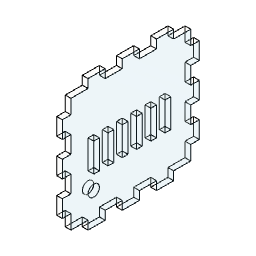
case_3_3mm (Autodesk Fusion 360 design; units mm, degrees)
Autodesk Fusion 360 part; units mm, degrees
sketch "スケッチ1" plane through (0, 0, 0) normal (1, 0, 0) x (0, 1, 0)
  line L0 (0, 0) -> (46, 0)
  line L1 (46, 0) -> (46, 44)
  line L2 (46, 44) -> (0, 44)
  line L3 (0, 44) -> (0, 0)
  dimension "d1" = 46
  dimension "d2" = 44
  constraint horizontal L0
  constraint vertical L1
  constraint horizontal L2
  constraint vertical L3
  constraint coincident L0.start L3.end
  measures "d1" distance of L0.start L0.end
  measures "d2" distance of L0.end L1.end
extrude "押し出し1" add sketch "スケッチ1" along normal blind 2
sketch "スケッチ2" plane through (2, 0, 0) normal (1, 0, 0) x (0, 1, 0)
  line L0 (0, 44) -> (0, 0)
  line L1 (0, 0) -> (46, 0)
  line L2 (46, 0) -> (46, 44)
  line L3 (46, 44) -> (0, 44)
  line L4 (0, 0) -> (8, 0)
  line L5 (8, 0) -> (8, 2)
  line L6 (8, 2) -> (0, 2)
  line L7 (0, 2) -> (0, 0)
  line L8 (14, 0) -> (20, 0)
  line L9 (20, 0) -> (20, 2)
  line L10 (20, 2) -> (14, 2)
  line L11 (14, 2) -> (14, 0)
  line L12 (26, 0) -> (32, 0)
  line L13 (32, 0) -> (32, 2)
  line L14 (32, 2) -> (26, 2)
  line L15 (26, 2) -> (26, 0)
  line L16 (46, 0) -> (38, 0)
  line L17 (38, 0) -> (38, 2)
  line L18 (38, 2) -> (46, 2)
  line L19 (46, 2) -> (46, 0)
  line L20 (32, 42) -> (32, 44)
  line L21 (32, 44) -> (26, 44)
  line L22 (20, 42) -> (20, 44)
  line L23 (38, 42) -> (38, 44)
  line L24 (38, 44) -> (46, 44)
  line L25 (46, 44) -> (46, 42)
  line L26 (0, 42) -> (8, 42)
  line L27 (26, 44) -> (26, 42)
  line L28 (8, 42) -> (8, 44)
  line L29 (8, 44) -> (0, 44)
  line L30 (0, 44) -> (0, 42)
  line L31 (20, 44) -> (14, 44)
  line L32 (26, 42) -> (32, 42)
  line L33 (46, 42) -> (38, 42)
  line L34 (14, 42) -> (20, 42)
  line L35 (14, 44) -> (14, 42)
  point P0 (0, 42)
  dimension "d5" = 8
  dimension "d6" = 2
  dimension "d7" = 6
  dimension "d8" = 2
  dimension "d9" = 6
  dimension "d10" = 6
  dimension "d11" = 2
  dimension "d12" = 6
  dimension "d13" = 6
  dimension "d14" = 2
  constraint horizontal L4
  constraint vertical L5
  constraint horizontal L6
  constraint vertical L7
  constraint coincident L0.end L1.start
  constraint horizontal L8
  constraint vertical L9
  constraint horizontal L10
  constraint vertical L11
  constraint coincident L1 L8.start
  constraint horizontal L12
  constraint vertical L13
  constraint horizontal L14
  constraint vertical L15
  constraint coincident L1 L12.start
  constraint horizontal L16
  constraint vertical L17
  constraint horizontal L18
  constraint vertical L19
  constraint coincident L1.end L2.start
  measures "d5" distance of L5.end L6.end
  measures "d6" distance of L0.end L6.end
  measures "d7" distance of L9.end L10.end
  measures "d8" distance of L8.start L10.end
  measures "d9" distance of L5 L11
  measures "d10" distance of L13.end L14.end
  measures "d11" distance of L12.start L14.end
  measures "d12" distance of L9 L15
  measures "d13" distance of L13 L17
  measures "d14" distance of L1.end L18.end
extrude "押し出し2" cut sketch "スケッチ2" against normal blind 2 contours L0 L3 L26 L28 L29 L30 | L0 L1 L4 L5 L6 L7 | L3 L22 L31 L34 L35 | L3 L20 L21 L27 L32 | L1 L8 L9 L10 L11 | L2 L3 L23 L24 L25 L33 | L1 L12 L13 L14 L15 | L1 L2 L16 L17 L18 L19
sketch "スケッチ3" plane through (2, 0, 0) normal (1, 0, 0) x (0, 1, 0)
  line L0 (8, 2) -> (8, 0)
  line L1 (8, 0) -> (14, 0)
  line L2 (14, 0) -> (14, 2)
  line L3 (14, 2) -> (20, 2)
  line L4 (20, 2) -> (20, 0)
  line L5 (20, 0) -> (26, 0)
  line L6 (26, 0) -> (26, 2)
  line L7 (26, 2) -> (32, 2)
  line L8 (32, 2) -> (32, 0)
  line L9 (32, 0) -> (38, 0)
  line L10 (38, 0) -> (38, 2)
  line L11 (38, 2) -> (46, 2)
  line L12 (46, 2) -> (46, 42)
  line L13 (46, 42) -> (38, 42)
  line L14 (38, 42) -> (38, 44)
  line L15 (38, 44) -> (32, 44)
  line L16 (32, 44) -> (32, 42)
  line L17 (32, 42) -> (26, 42)
  line L18 (26, 42) -> (26, 44)
  line L19 (26, 44) -> (20, 44)
  line L20 (20, 44) -> (20, 42)
  line L21 (20, 42) -> (14, 42)
  line L22 (14, 42) -> (14, 44)
  line L23 (14, 44) -> (8, 44)
  line L24 (8, 44) -> (8, 42)
  line L25 (8, 42) -> (0, 42)
  line L26 (0, 42) -> (0, 2)
  line L27 (0, 2) -> (8, 2)
  line L28 (0, 44) -> (2, 44)
  line L29 (2, 44) -> (2, 37)
  line L30 (2, 37) -> (0, 37)
  line L31 (0, 37) -> (0, 44)
  line L32 (2, 31) -> (0, 31)
  line L33 (0, 31) -> (0, 25)
  line L34 (0, 25) -> (2, 25)
  line L35 (2, 25) -> (2, 31)
  line L36 (2, 19) -> (0, 19)
  line L37 (0, 19) -> (0, 13)
  line L38 (0, 13) -> (2, 13)
  line L39 (2, 13) -> (2, 19)
  line L40 (2, 7) -> (0, 7)
  line L41 (0, 7) -> (0, 0)
  line L42 (0, 0) -> (2, 0)
  line L43 (2, 0) -> (2, 7)
  line L44 (46, 31) -> (44, 31)
  line L45 (46, 13) -> (46, 19)
  line L46 (44, 44) -> (46, 44)
  line L47 (44, 0) -> (46, 0)
  line L48 (44, 7) -> (44, 0)
  line L49 (44, 25) -> (46, 25)
  line L50 (46, 37) -> (44, 37)
  line L51 (44, 37) -> (44, 44)
  line L52 (44, 13) -> (46, 13)
  line L53 (44, 31) -> (44, 25)
  line L54 (46, 19) -> (44, 19)
  line L55 (44, 19) -> (44, 13)
  line L56 (46, 25) -> (46, 31)
  line L57 (46, 7) -> (44, 7)
  line L58 (46, 0) -> (46, 7)
  line L59 (46, 44) -> (46, 37)
  point P0 (44, 0)
  dimension "d21" = 2
  dimension "d22" = 7
  dimension "d23" = 2
  dimension "d24" = 6
  dimension "d25" = 6
  dimension "d26" = 6
  dimension "d27" = 6
  dimension "d28" = 2
  dimension "d29" = 6
  dimension "d30" = 7
  dimension "d31" = 2
  constraint horizontal L28
  constraint vertical L29
  constraint horizontal L30
  constraint vertical L31
  constraint horizontal L32
  constraint vertical L33
  constraint horizontal L34
  constraint vertical L35
  constraint coincident L26 L33.end
  constraint horizontal L36
  constraint vertical L37
  constraint horizontal L38
  constraint vertical L39
  constraint coincident L26 L37.end
  constraint horizontal L40
  constraint vertical L41
  constraint horizontal L42
  constraint vertical L43
  constraint coincident L41.end L42.start
  measures "d21" distance of L28.start L28.end
  measures "d22" distance of L28.start L30.end
  measures "d23" distance of L32.start L32.end
  measures "d24" distance of L32.end L33.end
  measures "d25" distance of L30 L32
  measures "d26" distance of L34 L36
  measures "d27" distance of L36.end L37.end
  measures "d28" distance of L36.start L36.end
  measures "d29" distance of L38 L40
  measures "d30" distance of L40.end L41.end
  measures "d31" distance of L40.start L40.end
extrude "押し出し3" cut sketch "スケッチ3" against normal blind 2 contours L27 L41 L42 L43 | L26 L27 L40 L41 L43 | L26 L36 L37 L38 L39 | L26 L32 L33 L34 L35 | L25 L26 L29 L30 L31 | L25 L28 L29 L31 | L11 L12 L48 L57 L58 | L11 L47 L48 L58 | L12 L45 L52 L54 L55 | L12 L44 L49 L53 L56 | L12 L13 L50 L51 L59 | L13 L46 L51 L59
sketch "スケッチ4" plane through (2, 0, 0) normal (1, 0, 0) x (0, 1, 0)
  line L0 (44, 19) -> (46, 19)
  line L1 (46, 19) -> (46, 25)
  line L2 (46, 25) -> (44, 25)
  line L3 (44, 25) -> (44, 31)
  line L4 (44, 31) -> (46, 31)
  line L5 (46, 31) -> (46, 37)
  line L6 (46, 37) -> (44, 37)
  line L7 (44, 37) -> (44, 42)
  line L8 (44, 42) -> (38, 42)
  line L9 (38, 42) -> (38, 44)
  line L10 (38, 44) -> (32, 44)
  line L11 (32, 44) -> (32, 42)
  line L12 (32, 42) -> (26, 42)
  line L13 (26, 42) -> (26, 44)
  line L14 (26, 44) -> (20, 44)
  line L15 (20, 44) -> (20, 42)
  line L16 (20, 42) -> (14, 42)
  line L17 (14, 42) -> (14, 44)
  line L18 (14, 44) -> (8, 44)
  line L19 (8, 44) -> (8, 42)
  line L20 (8, 42) -> (2, 42)
  line L21 (2, 42) -> (2, 37)
  line L22 (2, 37) -> (0, 37)
  line L23 (0, 37) -> (0, 31)
  line L24 (0, 31) -> (2, 31)
  line L25 (2, 31) -> (2, 25)
  line L26 (2, 25) -> (0, 25)
  line L27 (0, 25) -> (0, 19)
  line L28 (0, 19) -> (2, 19)
  line L29 (2, 19) -> (2, 13)
  line L30 (2, 13) -> (0, 13)
  line L31 (0, 13) -> (0, 7)
  line L32 (0, 7) -> (2, 7)
  line L33 (2, 7) -> (2, 2)
  line L34 (2, 2) -> (8, 2)
  line L35 (8, 2) -> (8, 0)
  line L36 (8, 0) -> (14, 0)
  line L37 (14, 0) -> (14, 2)
  line L38 (14, 2) -> (20, 2)
  line L39 (20, 2) -> (20, 0)
  line L40 (20, 0) -> (26, 0)
  line L41 (26, 0) -> (26, 2)
  line L42 (26, 2) -> (32, 2)
  line L43 (32, 2) -> (32, 0)
  line L44 (32, 0) -> (38, 0)
  line L45 (38, 0) -> (38, 2)
  line L46 (38, 2) -> (44, 2)
  line L47 (44, 2) -> (44, 7)
  line L48 (44, 7) -> (46, 7)
  line L49 (46, 7) -> (46, 13)
  line L50 (46, 13) -> (44, 13)
  line L51 (44, 13) -> (44, 19)
  line L52 (10, 15) -> (12, 15)
  line L53 (12, 15) -> (12, 25)
  line L54 (12, 25) -> (10, 25)
  line L55 (10, 25) -> (10, 15)
  line L56 (15, 15) -> (17, 15)
  line L57 (17, 15) -> (17, 25)
  line L58 (17, 25) -> (15, 25)
  line L59 (15, 25) -> (15, 15)
  line L60 (20, 15) -> (22, 15)
  line L61 (22, 15) -> (22, 25)
  line L62 (22, 25) -> (20, 25)
  line L63 (20, 25) -> (20, 15)
  line L64 (25, 15) -> (27, 15)
  line L65 (27, 15) -> (27, 25)
  line L66 (27, 25) -> (25, 25)
  line L67 (25, 25) -> (25, 15)
  line L68 (30, 15) -> (32, 15)
  line L69 (32, 15) -> (32, 25)
  line L70 (32, 25) -> (30, 25)
  line L71 (30, 25) -> (30, 15)
  line L72 (35, 15) -> (37, 15)
  line L73 (37, 15) -> (37, 25)
  line L74 (37, 25) -> (35, 25)
  line L75 (35, 25) -> (35, 15)
  constraint horizontal L52
  constraint vertical L53
  constraint horizontal L54
  constraint vertical L55
  constraint horizontal L56
  constraint vertical L57
  constraint horizontal L58
  constraint vertical L59
  constraint horizontal L60
  constraint vertical L61
  constraint horizontal L62
  constraint vertical L63
  constraint horizontal L64
  constraint vertical L65
  constraint horizontal L66
  constraint vertical L67
  constraint horizontal L68
  constraint vertical L69
  constraint horizontal L70
  constraint vertical L71
  constraint horizontal L72
  constraint vertical L73
  constraint horizontal L74
  constraint vertical L75
extrude "押し出し4" cut sketch "スケッチ4" against normal blind 2 contours L52 L53 L54 L55 | L56 L57 L58 L59 | L60 L61 L62 L63 | L64 L65 L66 L67 | L68 L69 L70 L71 | L72 L73 L74 L75
sketch "スケッチ5" plane through (2, 0, 0) normal (1, 0, 0) x (0, 1, 0)
  line L0 (37, 15) -> (35, 15)
  line L1 (35, 15) -> (35, 25)
  line L2 (35, 25) -> (37, 25)
  line L3 (37, 25) -> (37, 15)
  line L4 (32, 15) -> (30, 15)
  line L5 (30, 15) -> (30, 25)
  line L6 (30, 25) -> (32, 25)
  line L7 (32, 25) -> (32, 15)
  line L8 (17, 15) -> (15, 15)
  line L9 (15, 15) -> (15, 25)
  line L10 (15, 25) -> (17, 25)
  line L11 (17, 25) -> (17, 15)
  line L12 (12, 15) -> (10, 15)
  line L13 (10, 15) -> (10, 25)
  line L14 (10, 25) -> (12, 25)
  line L15 (12, 25) -> (12, 15)
  line L16 (22, 15) -> (20, 15)
  line L17 (20, 15) -> (20, 25)
  line L18 (20, 25) -> (22, 25)
  line L19 (22, 25) -> (22, 15)
  line L20 (27, 15) -> (25, 15)
  line L21 (25, 15) -> (25, 25)
  line L22 (25, 25) -> (27, 25)
  line L23 (27, 25) -> (27, 15)
  line L24 (44, 19) -> (46, 19)
  line L25 (46, 19) -> (46, 25)
  line L26 (46, 25) -> (44, 25)
  line L27 (44, 25) -> (44, 31)
  line L28 (44, 31) -> (46, 31)
  line L29 (46, 31) -> (46, 37)
  line L30 (46, 37) -> (44, 37)
  line L31 (44, 37) -> (44, 42)
  line L32 (44, 42) -> (38, 42)
  line L33 (38, 42) -> (38, 44)
  line L34 (38, 44) -> (32, 44)
  line L35 (32, 44) -> (32, 42)
  line L36 (32, 42) -> (26, 42)
  line L37 (26, 42) -> (26, 44)
  line L38 (26, 44) -> (20, 44)
  line L39 (20, 44) -> (20, 42)
  line L40 (20, 42) -> (14, 42)
  line L41 (14, 42) -> (14, 44)
  line L42 (14, 44) -> (8, 44)
  line L43 (8, 44) -> (8, 42)
  line L44 (8, 42) -> (2, 42)
  line L45 (2, 42) -> (2, 37)
  line L46 (2, 37) -> (0, 37)
  line L47 (0, 37) -> (0, 31)
  line L48 (0, 31) -> (2, 31)
  line L49 (2, 31) -> (2, 25)
  line L50 (2, 25) -> (0, 25)
  line L51 (0, 25) -> (0, 19)
  line L52 (0, 19) -> (2, 19)
  line L53 (2, 19) -> (2, 13)
  line L54 (2, 13) -> (0, 13)
  line L55 (0, 13) -> (0, 7)
  line L56 (0, 7) -> (2, 7)
  line L57 (2, 7) -> (2, 2)
  line L58 (2, 2) -> (8, 2)
  line L59 (8, 2) -> (8, 0)
  line L60 (8, 0) -> (14, 0)
  line L61 (14, 0) -> (14, 2)
  line L62 (14, 2) -> (20, 2)
  line L63 (20, 2) -> (20, 0)
  line L64 (20, 0) -> (26, 0)
  line L65 (26, 0) -> (26, 2)
  line L66 (26, 2) -> (32, 2)
  line L67 (32, 2) -> (32, 0)
  line L68 (32, 0) -> (38, 0)
  line L69 (38, 0) -> (38, 2)
  line L70 (38, 2) -> (44, 2)
  line L71 (44, 2) -> (44, 7)
  line L72 (44, 7) -> (46, 7)
  line L73 (46, 7) -> (46, 13)
  line L74 (46, 13) -> (44, 13)
  line L75 (44, 13) -> (44, 19)
  circle A0 centre (10, 10) radius 2
extrude "押し出し5" cut sketch "スケッチ5" against normal blind 2 contours A0
sketch "スケッチ6" plane through (2, 0, 0) normal (1, 0, 0) x (0, 1, 0)
  circle A0 centre (10, 10) radius 2
  line L0 (37, 15) -> (35, 15)
  line L1 (35, 15) -> (35, 25)
  line L2 (35, 25) -> (37, 25)
  line L3 (37, 25) -> (37, 15)
  line L4 (32, 15) -> (30, 15)
  line L5 (30, 15) -> (30, 25)
  line L6 (30, 25) -> (32, 25)
  line L7 (32, 25) -> (32, 15)
  line L8 (17, 15) -> (15, 15)
  line L9 (15, 15) -> (15, 25)
  line L10 (15, 25) -> (17, 25)
  line L11 (17, 25) -> (17, 15)
  line L12 (12, 15) -> (10, 15)
  line L13 (10, 15) -> (10, 25)
  line L14 (10, 25) -> (12, 25)
  line L15 (12, 25) -> (12, 15)
  line L16 (22, 15) -> (20, 15)
  line L17 (20, 15) -> (20, 25)
  line L18 (20, 25) -> (22, 25)
  line L19 (22, 25) -> (22, 15)
  line L20 (27, 15) -> (25, 15)
  line L21 (25, 15) -> (25, 25)
  line L22 (25, 25) -> (27, 25)
  line L23 (27, 25) -> (27, 15)
  line L24 (44, 19) -> (46, 19)
  line L25 (46, 19) -> (46, 25)
  line L26 (46, 25) -> (44, 25)
  line L27 (44, 25) -> (44, 31)
  line L28 (44, 31) -> (46, 31)
  line L29 (46, 31) -> (46, 37)
  line L30 (46, 37) -> (44, 37)
  line L31 (44, 37) -> (44, 42)
  line L32 (44, 42) -> (38, 42)
  line L33 (38, 42) -> (38, 44)
  line L34 (38, 44) -> (32, 44)
  line L35 (32, 44) -> (32, 42)
  line L36 (32, 42) -> (26, 42)
  line L37 (26, 42) -> (26, 44)
  line L38 (26, 44) -> (20, 44)
  line L39 (20, 44) -> (20, 42)
  line L40 (20, 42) -> (14, 42)
  line L41 (14, 42) -> (14, 44)
  line L42 (14, 44) -> (8, 44)
  line L43 (8, 44) -> (8, 42)
  line L44 (8, 42) -> (2, 42)
  line L45 (2, 42) -> (2, 37)
  line L46 (2, 37) -> (0, 37)
  line L47 (0, 37) -> (0, 31)
  line L48 (0, 31) -> (2, 31)
  line L49 (2, 31) -> (2, 25)
  line L50 (2, 25) -> (0, 25)
  line L51 (0, 25) -> (0, 19)
  line L52 (0, 19) -> (2, 19)
  line L53 (2, 19) -> (2, 13)
  line L54 (2, 13) -> (0, 13)
  line L55 (0, 13) -> (0, 7)
  line L56 (0, 7) -> (2, 7)
  line L57 (2, 7) -> (2, 2)
  line L58 (2, 2) -> (8, 2)
  line L59 (8, 2) -> (8, 0)
  line L60 (8, 0) -> (14, 0)
  line L61 (14, 0) -> (14, 2)
  line L62 (14, 2) -> (20, 2)
  line L63 (20, 2) -> (20, 0)
  line L64 (20, 0) -> (26, 0)
  line L65 (26, 0) -> (26, 2)
  line L66 (26, 2) -> (32, 2)
  line L67 (32, 2) -> (32, 0)
  line L68 (32, 0) -> (38, 0)
  line L69 (38, 0) -> (38, 2)
  line L70 (38, 2) -> (44, 2)
  line L71 (44, 2) -> (44, 7)
  line L72 (44, 7) -> (46, 7)
  line L73 (46, 7) -> (46, 13)
  line L74 (46, 13) -> (44, 13)
  line L75 (44, 13) -> (44, 19)
  line L76 (8, 44) -> (14, 44)
  line L77 (14, 44) -> (14, 45)
  line L78 (14, 45) -> (8, 45)
  line L79 (8, 45) -> (8, 44)
  line L80 (20, 44) -> (26, 44)
  line L81 (26, 44) -> (26, 45)
  line L82 (26, 45) -> (20, 45)
  line L83 (20, 45) -> (20, 44)
  line L84 (32, 44) -> (38, 44)
  line L85 (38, 44) -> (38, 45)
  line L86 (38, 45) -> (32, 45)
  line L87 (32, 45) -> (32, 44)
  line L88 (46, 37) -> (47, 37)
  line L89 (47, 37) -> (47, 31)
  line L90 (47, 31) -> (46, 31)
  line L91 (46, 31) -> (46, 37)
  line L92 (46, 25) -> (47, 25)
  line L93 (47, 25) -> (47, 19)
  line L94 (47, 19) -> (46, 19)
  line L95 (46, 19) -> (46, 25)
  line L96 (46, 13) -> (47, 13)
  line L97 (47, 13) -> (47, 7)
  line L98 (47, 7) -> (46, 7)
  line L99 (46, 7) -> (46, 13)
  line L100 (38, 0) -> (32, 0)
  line L101 (32, 0) -> (32, -1)
  line L102 (32, -1) -> (38, -1)
  line L103 (38, -1) -> (38, 0)
  line L104 (26, 0) -> (20, 0)
  line L105 (20, 0) -> (20, -1)
  line L106 (20, -1) -> (26, -1)
  line L107 (26, -1) -> (26, 0)
  line L108 (14, 0) -> (8, 0)
  line L109 (8, 0) -> (8, -1)
  line L110 (8, -1) -> (14, -1)
  line L111 (14, -1) -> (14, 0)
  line L112 (-1, 7) -> (0, 7)
  line L113 (0, 7) -> (0, 13)
  line L114 (0, 13) -> (-1, 13)
  line L115 (-1, 13) -> (-1, 7)
  line L116 (-1, 19) -> (0, 19)
  line L117 (0, 19) -> (0, 25)
  line L118 (0, 25) -> (-1, 25)
  line L119 (-1, 25) -> (-1, 19)
  line L120 (-1, 31) -> (0, 31)
  line L121 (0, 31) -> (0, 37)
  line L122 (0, 37) -> (-1, 37)
  line L123 (-1, 37) -> (-1, 31)
  constraint horizontal L76
  constraint vertical L77
  constraint horizontal L78
  constraint vertical L79
  constraint coincident L42.end L43.start
  constraint horizontal L80
  constraint vertical L81
  constraint horizontal L82
  constraint vertical L83
  constraint coincident L38.end L39.start
  constraint horizontal L84
  constraint vertical L85
  constraint horizontal L86
  constraint vertical L87
  constraint coincident L34.end L35.start
  constraint horizontal L88
  constraint vertical L89
  constraint horizontal L90
  constraint vertical L91
  constraint coincident L29.end L30.start
  constraint horizontal L92
  constraint vertical L93
  constraint horizontal L94
  constraint vertical L95
  constraint coincident L25.end L26.start
  constraint horizontal L96
  constraint vertical L97
  constraint horizontal L98
  constraint vertical L99
  constraint coincident L73.end L74.start
  constraint horizontal L100
  constraint vertical L101
  constraint horizontal L102
  constraint vertical L103
  constraint coincident L68.end L69.start
  constraint horizontal L104
  constraint vertical L105
  constraint horizontal L106
  constraint vertical L107
  constraint coincident L64.end L65.start
  constraint horizontal L108
  constraint vertical L109
  constraint horizontal L110
  constraint vertical L111
  constraint coincident L60.end L61.start
  constraint horizontal L112
  constraint vertical L113
  constraint horizontal L114
  constraint vertical L115
  constraint coincident L54.end L55.start
  constraint horizontal L116
  constraint vertical L117
  constraint horizontal L118
  constraint vertical L119
  constraint coincident L50.end L51.start
  constraint horizontal L120
  constraint vertical L121
  constraint horizontal L122
  constraint vertical L123
  constraint coincident L46.end L47.start
extrude "押し出し6" add sketch "スケッチ6" against normal blind 2 contours L25 L92 L93 L94 L95 | L73 L96 L97 L98 L99 | L29 L88 L89 L90 L91 | L68 L100 L101 L102 L103 | L34 L84 L85 L86 L87 | L64 L104 L105 L106 L107 | L38 L80 L81 L82 L83 | L60 L108 L109 L110 L111 | L42 L76 L77 L78 L79 | L55 L112 L113 L114 L115 | L47 L120 L121 L122 L123 | L51 L116 L117 L118 L119
sketch "スケッチ7" plane through (2, 0, 0) normal (1, 0, 0) x (0, 1, 0)
  circle A0 centre (10, 10) radius 2
  line L0 (37, 15) -> (35, 15)
  line L1 (35, 15) -> (35, 25)
  line L2 (35, 25) -> (37, 25)
  line L3 (37, 25) -> (37, 15)
  line L4 (32, 15) -> (30, 15)
  line L5 (30, 15) -> (30, 25)
  line L6 (30, 25) -> (32, 25)
  line L7 (32, 25) -> (32, 15)
  line L8 (17, 15) -> (15, 15)
  line L9 (15, 15) -> (15, 25)
  line L10 (15, 25) -> (17, 25)
  line L11 (17, 25) -> (17, 15)
  line L12 (12, 15) -> (10, 15)
  line L13 (10, 15) -> (10, 25)
  line L14 (10, 25) -> (12, 25)
  line L15 (12, 25) -> (12, 15)
  line L16 (22, 15) -> (20, 15)
  line L17 (20, 15) -> (20, 25)
  line L18 (20, 25) -> (22, 25)
  line L19 (22, 25) -> (22, 15)
  line L20 (27, 15) -> (25, 15)
  line L21 (25, 15) -> (25, 25)
  line L22 (25, 25) -> (27, 25)
  line L23 (27, 25) -> (27, 15)
  line L24 (44, 19) -> (47, 19)
  line L25 (47, 19) -> (47, 25)
  line L26 (47, 25) -> (44, 25)
  line L27 (44, 25) -> (44, 31)
  line L28 (44, 31) -> (47, 31)
  line L29 (47, 31) -> (47, 37)
  line L30 (47, 37) -> (44, 37)
  line L31 (44, 37) -> (44, 42)
  line L32 (44, 42) -> (38, 42)
  line L33 (38, 42) -> (38, 45)
  line L34 (38, 45) -> (32, 45)
  line L35 (32, 45) -> (32, 42)
  line L36 (32, 42) -> (26, 42)
  line L37 (26, 42) -> (26, 45)
  line L38 (26, 45) -> (20, 45)
  line L39 (20, 45) -> (20, 42)
  line L40 (20, 42) -> (14, 42)
  line L41 (14, 42) -> (14, 45)
  line L42 (14, 45) -> (8, 45)
  line L43 (8, 45) -> (8, 42)
  line L44 (8, 42) -> (2, 42)
  line L45 (2, 42) -> (2, 37)
  line L46 (2, 37) -> (-1, 37)
  line L47 (-1, 37) -> (-1, 31)
  line L48 (-1, 31) -> (2, 31)
  line L49 (2, 31) -> (2, 25)
  line L50 (2, 25) -> (-1, 25)
  line L51 (-1, 25) -> (-1, 19)
  line L52 (-1, 19) -> (2, 19)
  line L53 (2, 19) -> (2, 13)
  line L54 (2, 13) -> (-1, 13)
  line L55 (-1, 13) -> (-1, 7)
  line L56 (-1, 7) -> (2, 7)
  line L57 (2, 7) -> (2, 2)
  line L58 (2, 2) -> (8, 2)
  line L59 (8, 2) -> (8, -1)
  line L60 (8, -1) -> (14, -1)
  line L61 (14, -1) -> (14, 2)
  line L62 (14, 2) -> (20, 2)
  line L63 (20, 2) -> (20, -1)
  line L64 (20, -1) -> (26, -1)
  line L65 (26, -1) -> (26, 2)
  line L66 (26, 2) -> (32, 2)
  line L67 (32, 2) -> (32, -1)
  line L68 (32, -1) -> (38, -1)
  line L69 (38, -1) -> (38, 2)
  line L70 (38, 2) -> (44, 2)
  line L71 (44, 2) -> (44, 7)
  line L72 (44, 7) -> (47, 7)
  line L73 (47, 7) -> (47, 13)
  line L74 (47, 13) -> (44, 13)
  line L75 (44, 13) -> (44, 19)
